Autodesk Inventor part; units mm, degrees
(part 4 of 4)
sketch "Sketch14" plane through (0, 0, 3) normal (0, 0, 1) x (1, 0, 0)
  line L0 (-25.3933, -129) -> (-25.3933, -146.5) projected
  line L1 (-25.3933, -146.5) -> (23.6067, -146.5) projected
  line L2 (23.6067, -146.5) -> (23.6067, -129) projected
  line L3 (23.6067, -129) -> (100.5, -129) projected
  line L4 (100.5, -129) -> (100.5, 184.5) projected
  line L5 (100.5, 184.5) -> (81, 184.5) projected
  line L6 (81, 184.5) -> (81, 215) projected
  line L7 (81, 215) -> (-78, 215) projected
  line L8 (-78, 215) -> (-78, 46.0635) projected
  line L9 (-78, 46.0635) -> (-75, 46.0635) projected
  line L10 (-75, 46.0635) -> (-75, 40.8932) projected
  line L11 (-75, 40.8932) -> (-78, 40.8932) projected
  line L12 (-78, 40.8932) -> (-78, 30.6062) projected
  line L13 (-78, 30.6062) -> (-75, 30.6062) projected
  line L14 (-75, 30.6062) -> (-75, 20.5478) projected
  line L15 (-75, 20.5478) -> (-78, 20.5478) projected
  line L16 (-78, 20.5478) -> (-78, 10.2608) projected
  line L17 (-78, 10.2608) -> (-75, 10.2608) projected
  line L18 (-75, 10.2608) -> (-75, -0.1068) projected
  line L19 (-75, -0.1068) -> (-78, -0.1068) projected
  line L20 (-78, -0.1068) -> (-78, -10.3938) projected
  line L21 (-78, -10.3938) -> (-75, -10.3938) projected
  line L22 (-75, -10.3938) -> (-75, -20.4522) projected
  line L23 (-75, -20.4522) -> (-78, -20.4522) projected
  line L24 (-78, -20.4522) -> (-78, -30.7392) projected
  line L25 (-78, -30.7392) -> (-75, -30.7392) projected
  line L26 (-75, -30.7392) -> (-75, -41.1068) projected
  line L27 (-75, -41.1068) -> (-78, -41.1068) projected
  line L28 (-78, -41.1068) -> (-78, -51.3938) projected
  line L29 (-78, -51.3938) -> (-75, -51.3938) projected
  line L30 (-75, -51.3938) -> (-75, -61.4522) projected
  line L31 (-75, -61.4522) -> (-78, -61.4522) projected
  line L32 (-78, -61.4522) -> (-78, -71.7392) projected
  line L33 (-78, -71.7392) -> (-75, -71.7392) projected
  line L34 (-75, -71.7392) -> (-75, -82.1068) projected
  line L35 (-75, -82.1068) -> (-78, -82.1068) projected
  line L36 (-78, -82.1068) -> (-78, -92.3938) projected
  line L37 (-78, -92.3938) -> (-75, -92.3938) projected
  line L38 (-75, -92.3938) -> (-75, -102.4522) projected
  line L39 (-75, -102.4522) -> (-78, -102.4522) projected
  line L40 (-78, -102.4522) -> (-78, -112.7392) projected
  line L41 (-78, -112.7392) -> (-75, -112.7392) projected
  line L42 (-75, -112.7392) -> (-75, -129) projected
  line L43 (-75, -129) -> (-25.3933, -129) projected
  arc A0 (46.9188, 54.6398) -> (53.7912, 60.27) centre (23.569, 90.1509) ccw projected
  arc A1 (35.9306, 51.3509) -> (46.9188, 54.6398) centre (35.9306, 71.3509) ccw projected
  line L44 (35.9306, 51.3509) -> (11.2074, 51.3509) projected
  arc A2 (0.2192, 54.6398) -> (11.2074, 51.3509) centre (11.2074, 71.3509) ccw projected
  arc A3 (-6.6532, 60.27) -> (0.2192, 54.6398) centre (23.569, 90.1509) ccw projected
  arc A4 (-12.431, 74.3316) -> (-6.6532, 60.27) centre (7.569, 74.3316) ccw projected
  line L45 (-12.431, 74.3316) -> (-12.431, 105.9702) projected
  arc A5 (-6.6532, 120.0317) -> (-12.431, 105.9702) centre (7.569, 105.9702) ccw projected
  arc A6 (0.2192, 125.662) -> (-6.6532, 120.0317) centre (23.569, 90.1509) ccw projected
  arc A7 (11.2074, 128.9509) -> (0.2192, 125.662) centre (11.2074, 108.9509) ccw projected
  line L46 (11.2074, 128.9509) -> (35.9306, 128.9509) projected
  arc A8 (46.9188, 125.662) -> (35.9306, 128.9509) centre (35.9306, 108.9509) ccw projected
  arc A9 (53.7912, 120.0317) -> (46.9188, 125.662) centre (23.569, 90.1509) ccw projected
  arc A10 (59.569, 105.9702) -> (53.7912, 120.0317) centre (39.569, 105.9702) ccw projected
  line L47 (59.569, 105.9702) -> (59.569, 74.3316) projected
  arc A11 (53.7912, 60.27) -> (59.569, 74.3316) centre (39.569, 74.3316) ccw projected
  circle A12 centre (-12.181, 208.9009) radius 1.2 projected
  circle A13 centre (59.319, 137.4009) radius 1.2 projected
  circle A14 centre (-12.181, 137.4009) radius 1.2 projected
  circle A15 centre (59.319, 54.4009) radius 1.2 projected
  circle A16 centre (-12.181, 125.9009) radius 1.2 projected
  circle A17 centre (59.319, 125.9009) radius 1.2 projected
  circle A18 centre (59.319, 208.9009) radius 1.2 projected
  circle A19 centre (-12.181, 54.4009) radius 1.2 projected
  arc A20 (46.9188, 137.6398) -> (53.7912, 143.27) centre (23.569, 173.1509) ccw projected
  arc A21 (35.9306, 134.3509) -> (46.9188, 137.6398) centre (35.9306, 154.3509) ccw projected
  line L48 (35.9306, 134.3509) -> (11.2074, 134.3509) projected
  arc A22 (0.2192, 137.6398) -> (11.2074, 134.3509) centre (11.2074, 154.3509) ccw projected
  arc A23 (-6.6532, 143.27) -> (0.2192, 137.6398) centre (23.569, 173.1509) ccw projected
  arc A24 (-12.431, 157.3316) -> (-6.6532, 143.27) centre (7.569, 157.3316) ccw projected
  line L49 (-12.431, 157.3316) -> (-12.431, 188.9702) projected
  arc A25 (-6.6532, 203.0317) -> (-12.431, 188.9702) centre (7.569, 188.9702) ccw projected
  arc A26 (0.2192, 208.662) -> (-6.6532, 203.0317) centre (23.569, 173.1509) ccw projected
  arc A27 (11.2074, 211.9509) -> (0.2192, 208.662) centre (11.2074, 191.9509) ccw projected
  line L50 (11.2074, 211.9509) -> (35.9306, 211.9509) projected
  arc A28 (46.9188, 208.662) -> (35.9306, 211.9509) centre (35.9306, 191.9509) ccw projected
  arc A29 (53.7912, 203.0317) -> (46.9188, 208.662) centre (23.569, 173.1509) ccw projected
  arc A30 (59.569, 188.9702) -> (53.7912, 203.0317) centre (39.569, 188.9702) ccw projected
  line L51 (59.569, 188.9702) -> (59.569, 157.3316) projected
  arc A31 (53.7912, 143.27) -> (59.569, 157.3316) centre (39.569, 157.3316) ccw projected
  circle A32 centre (90.5, 174.5) radius 2.25 projected
  circle A33 centre (90.5, 131.8987) radius 2.25 projected
  circle A34 centre (90.5, 58.3987) radius 2.25 projected
  circle A35 centre (90.5, -117.6237) radius 2.25 projected
  circle A36 centre (-17.8933, -140) radius 2.25 projected
  circle A37 centre (16.1067, -140) radius 2.25 projected
  line L52 (-58.9404, 10.4643) -> (-58.9404, 20.3443) projected
  arc A38 (-55.9404, 23.3443) -> (-58.9404, 20.3443) centre (-55.9404, 20.3443) ccw projected
  line L53 (-55.9404, 23.3443) -> (31.7396, 23.3443) projected
  arc A39 (34.7396, 20.3443) -> (31.7396, 23.3443) centre (31.7396, 20.3443) ccw projected
  line L54 (34.7396, 20.3443) -> (34.7396, 10.4643) projected
  arc A40 (31.7396, 7.4643) -> (34.7396, 10.4643) centre (31.7396, 10.4643) ccw projected
  line L55 (31.7396, 7.4643) -> (-55.9404, 7.4643) projected
  arc A41 (-58.9404, 10.4643) -> (-55.9404, 7.4643) centre (-55.9404, 10.4643) ccw projected
  line L56 (-58.9404, 30.8097) -> (-58.9404, 40.6897) projected
  arc A42 (-55.9404, 43.6897) -> (-58.9404, 40.6897) centre (-55.9404, 40.6897) ccw projected
  line L57 (-55.9404, 43.6897) -> (31.7396, 43.6897) projected
  arc A43 (34.7396, 40.6897) -> (31.7396, 43.6897) centre (31.7396, 40.6897) ccw projected
  line L58 (34.7396, 40.6897) -> (34.7396, 30.8097) projected
  arc A44 (31.7396, 27.8097) -> (34.7396, 30.8097) centre (31.7396, 30.8097) ccw projected
  line L59 (31.7396, 27.8097) -> (-55.9404, 27.8097) projected
  arc A45 (-58.9404, 30.8097) -> (-55.9404, 27.8097) centre (-55.9404, 30.8097) ccw projected
  arc A46 (-55.9404, 2.9989) -> (-58.9404, -0.0011) centre (-55.9404, -0.0011) ccw projected
  line L60 (-55.9404, 2.9989) -> (31.7396, 2.9989) projected
  arc A47 (34.7396, -0.0011) -> (31.7396, 2.9989) centre (31.7396, -0.0011) ccw projected
  line L61 (34.7396, -0.0011) -> (34.7396, -9.8811) projected
  arc A48 (31.7396, -12.8811) -> (34.7396, -9.8811) centre (31.7396, -9.8811) ccw projected
  line L62 (31.7396, -12.8811) -> (-55.9404, -12.8811) projected
  arc A49 (-58.9404, -9.8811) -> (-55.9404, -12.8811) centre (-55.9404, -9.8811) ccw projected
  line L63 (-58.9404, -9.8811) -> (-58.9404, -0.0011) projected
  arc A50 (-55.9404, -37.6919) -> (-58.9404, -40.6919) centre (-55.9404, -40.6919) ccw projected
  line L64 (-55.9404, -37.6919) -> (31.7396, -37.6919) projected
  arc A51 (34.7396, -40.6919) -> (31.7396, -37.6919) centre (31.7396, -40.6919) ccw projected
  line L65 (34.7396, -40.6919) -> (34.7396, -50.5719) projected
  arc A52 (31.7396, -53.5719) -> (34.7396, -50.5719) centre (31.7396, -50.5719) ccw projected
  line L66 (31.7396, -53.5719) -> (-55.9404, -53.5719) projected
  arc A53 (-58.9404, -50.5719) -> (-55.9404, -53.5719) centre (-55.9404, -50.5719) ccw projected
  line L67 (-58.9404, -50.5719) -> (-58.9404, -40.6919) projected
  line L68 (-55.9404, -58.0373) -> (31.7396, -58.0373) projected
  arc A54 (34.7396, -61.0373) -> (31.7396, -58.0373) centre (31.7396, -61.0373) ccw projected
  line L69 (34.7396, -61.0373) -> (34.7396, -70.9173) projected
  arc A55 (31.7396, -73.9173) -> (34.7396, -70.9173) centre (31.7396, -70.9173) ccw projected
  line L70 (31.7396, -73.9173) -> (-55.9404, -73.9173) projected
  arc A56 (-58.9404, -70.9173) -> (-55.9404, -73.9173) centre (-55.9404, -70.9173) ccw projected
  line L71 (-58.9404, -70.9173) -> (-58.9404, -61.0373) projected
  arc A57 (-55.9404, -58.0373) -> (-58.9404, -61.0373) centre (-55.9404, -61.0373) ccw projected
  line L72 (31.7396, -33.2265) -> (-55.9404, -33.2265) projected
  arc A58 (-58.9404, -30.2265) -> (-55.9404, -33.2265) centre (-55.9404, -30.2265) ccw projected
  line L73 (-58.9404, -30.2265) -> (-58.9404, -20.3465) projected
  arc A59 (-55.9404, -17.3465) -> (-58.9404, -20.3465) centre (-55.9404, -20.3465) ccw projected
  line L74 (-55.9404, -17.3465) -> (31.7396, -17.3465) projected
  arc A60 (34.7396, -20.3465) -> (31.7396, -17.3465) centre (31.7396, -20.3465) ccw projected
  line L75 (34.7396, -20.3465) -> (34.7396, -30.2265) projected
  arc A61 (31.7396, -33.2265) -> (34.7396, -30.2265) centre (31.7396, -30.2265) ccw projected
  arc A62 (34.7396, -81.3827) -> (31.7396, -78.3827) centre (31.7396, -81.3827) ccw projected
  line L76 (34.7396, -81.3827) -> (34.7396, -91.2627) projected
  arc A63 (31.7396, -94.2627) -> (34.7396, -91.2627) centre (31.7396, -91.2627) ccw projected
  line L77 (31.7396, -94.2627) -> (-55.9404, -94.2627) projected
  arc A64 (-58.9404, -91.2627) -> (-55.9404, -94.2627) centre (-55.9404, -91.2627) ccw projected
  line L78 (-58.9404, -91.2627) -> (-58.9404, -81.3827) projected
  arc A65 (-55.9404, -78.3827) -> (-58.9404, -81.3827) centre (-55.9404, -81.3827) ccw projected
  line L79 (-55.9404, -78.3827) -> (31.7396, -78.3827) projected
  arc A66 (31.7396, -114.6081) -> (34.7396, -111.6081) centre (31.7396, -111.6081) ccw projected
  line L80 (31.7396, -114.6081) -> (-55.9404, -114.6081) projected
  arc A67 (-58.9404, -111.6081) -> (-55.9404, -114.6081) centre (-55.9404, -111.6081) ccw projected
  line L81 (-58.9404, -111.6081) -> (-58.9404, -101.7281) projected
  arc A68 (-55.9404, -98.7281) -> (-58.9404, -101.7281) centre (-55.9404, -101.7281) ccw projected
  line L82 (-55.9404, -98.7281) -> (31.7396, -98.7281) projected
  arc A69 (34.7396, -101.7281) -> (31.7396, -98.7281) centre (31.7396, -101.7281) ccw projected
  line L83 (34.7396, -101.7281) -> (34.7396, -111.6081) projected
  line L84 (-69.3194, 50.0635) -> (-69.3194, 207.0635) projected
  arc A70 (-68.3194, 208.0635) -> (-69.3194, 207.0635) centre (-68.3194, 207.0635) ccw projected
  line L85 (-68.3194, 208.0635) -> (-25.6194, 208.0635) projected
  arc A71 (-24.6194, 207.0635) -> (-25.6194, 208.0635) centre (-25.6194, 207.0635) ccw projected
  line L86 (-24.6194, 207.0635) -> (-24.6194, 50.0635) projected
  arc A72 (-25.6194, 49.0635) -> (-24.6194, 50.0635) centre (-25.6194, 50.0635) ccw projected
  line L87 (-25.6194, 49.0635) -> (-68.3194, 49.0635) projected
  arc A73 (-69.3194, 50.0635) -> (-68.3194, 49.0635) centre (-68.3194, 50.0635) ccw projected
  line L88 (64, 48.3987) -> (64, -109.7094) projected
  arc A74 (63.7071, -110.4166) -> (64, -109.7094) centre (63, -109.7094) ccw projected
  line L89 (63.7071, -110.4166) -> (59.2929, -114.8308) projected
  arc A75 (58.5858, -115.1237) -> (59.2929, -114.8308) centre (58.5858, -114.1237) ccw projected
  line L90 (58.5858, -115.1237) -> (43.2196, -115.1237) projected
  arc A76 (42.2196, -114.1237) -> (43.2196, -115.1237) centre (43.2196, -114.1237) ccw projected
  line L91 (42.2196, -114.1237) -> (42.2196, -104.6674) projected
  arc A77 (42.2196, -104.6674) -> (40.773, -102.7455) centre (40.2196, -104.6674) ccw projected
  arc A78 (39.7673, -102.1811) -> (40.773, -102.7455) centre (41.4696, -100.3262) ccw projected
  arc A79 (39.1196, -100.7076) -> (39.7673, -102.1811) centre (41.1196, -100.7076) ccw projected
  line L92 (39.1196, -100.7076) -> (39.1196, -95.7515) projected
  arc A80 (39.7673, -94.2779) -> (39.1196, -95.7515) centre (41.1196, -95.7515) ccw projected
  arc A81 (39.937, -94.1354) -> (39.7673, -94.2779) centre (41.4696, -96.1328) ccw projected
  arc A82 (39.937, -94.1354) -> (40.7196, -92.5486) centre (38.7196, -92.5486) ccw projected
  line L93 (40.7196, -92.5486) -> (40.7196, -83.4104) projected
  arc A83 (40.7196, -83.4104) -> (39.937, -81.8236) centre (38.7196, -83.4104) ccw projected
  arc A84 (39.7673, -81.6811) -> (39.937, -81.8236) centre (41.4696, -79.8262) ccw projected
  arc A85 (39.1196, -80.2076) -> (39.7673, -81.6811) centre (41.1196, -80.2076) ccw projected
  line L94 (39.1196, -80.2076) -> (39.1196, -75.2515) projected
  arc A86 (39.7673, -73.7779) -> (39.1196, -75.2515) centre (41.1196, -75.2515) ccw projected
  arc A87 (39.937, -73.6354) -> (39.7673, -73.7779) centre (41.4696, -75.6328) ccw projected
  arc A88 (39.937, -73.6354) -> (40.7196, -72.0486) centre (38.7196, -72.0486) ccw projected
  line L95 (40.7196, -72.0486) -> (40.7196, -62.9104) projected
  arc A89 (40.7196, -62.9104) -> (39.937, -61.3236) centre (38.7196, -62.9104) ccw projected
  arc A90 (39.7673, -61.1811) -> (39.937, -61.3236) centre (41.4696, -59.3262) ccw projected
  arc A91 (39.1196, -59.7076) -> (39.7673, -61.1811) centre (41.1196, -59.7076) ccw projected
  line L96 (39.1196, -59.7076) -> (39.1196, -54.7515) projected
  arc A92 (39.7673, -53.2779) -> (39.1196, -54.7515) centre (41.1196, -54.7515) ccw projected
  arc A93 (39.937, -53.1354) -> (39.7673, -53.2779) centre (41.4696, -55.1328) ccw projected
  arc A94 (39.937, -53.1354) -> (40.7196, -51.5486) centre (38.7196, -51.5486) ccw projected
  line L97 (40.7196, -51.5486) -> (40.7196, -42.4104) projected
  arc A95 (40.7196, -42.4104) -> (39.937, -40.8236) centre (38.7196, -42.4104) ccw projected
  arc A96 (39.7673, -40.6811) -> (39.937, -40.8236) centre (41.4696, -38.8262) ccw projected
  arc A97 (39.1196, -39.2076) -> (39.7673, -40.6811) centre (41.1196, -39.2076) ccw projected
  line L98 (39.1196, -39.2076) -> (39.1196, -34.2515) projected
  arc A98 (39.7673, -32.7779) -> (39.1196, -34.2515) centre (41.1196, -34.2515) ccw projected
  arc A99 (39.937, -32.6354) -> (39.7673, -32.7779) centre (41.4696, -34.6328) ccw projected
  arc A100 (39.937, -32.6354) -> (40.7196, -31.0486) centre (38.7196, -31.0486) ccw projected
  line L99 (40.7196, -31.0486) -> (40.7196, -21.9104) projected
  arc A101 (40.7196, -21.9104) -> (39.937, -20.3236) centre (38.7196, -21.9104) ccw projected
  arc A102 (39.7673, -20.1811) -> (39.937, -20.3236) centre (41.4696, -18.3262) ccw projected
  arc A103 (39.1196, -18.7076) -> (39.7673, -20.1811) centre (41.1196, -18.7076) ccw projected
  line L100 (39.1196, -18.7076) -> (39.1196, -13.7515) projected
  arc A104 (39.7673, -12.2779) -> (39.1196, -13.7515) centre (41.1196, -13.7515) ccw projected
  arc A105 (39.937, -12.1354) -> (39.7673, -12.2779) centre (41.4696, -14.1328) ccw projected
  arc A106 (39.937, -12.1354) -> (40.7196, -10.5486) centre (38.7196, -10.5486) ccw projected
  line L101 (40.7196, -10.5486) -> (40.7196, -1.4104) projected
  arc A107 (40.7196, -1.4104) -> (39.937, 0.1764) centre (38.7196, -1.4104) ccw projected
  arc A108 (39.7673, 0.3189) -> (39.937, 0.1764) centre (41.4696, 2.1738) ccw projected
  arc A109 (39.1196, 1.7924) -> (39.7673, 0.3189) centre (41.1196, 1.7924) ccw projected
  line L102 (39.1196, 1.7924) -> (39.1196, 6.7485) projected
  arc A110 (39.7673, 8.2221) -> (39.1196, 6.7485) centre (41.1196, 6.7485) ccw projected
  arc A111 (39.937, 8.3646) -> (39.7673, 8.2221) centre (41.4696, 6.3672) ccw projected
  arc A112 (39.937, 8.3646) -> (40.7196, 9.9514) centre (38.7196, 9.9514) ccw projected
  line L103 (40.7196, 9.9514) -> (40.7196, 19.0896) projected
  arc A113 (40.7196, 19.0896) -> (39.937, 20.6764) centre (38.7196, 19.0896) ccw projected
  arc A114 (39.7673, 20.8189) -> (39.937, 20.6764) centre (41.4696, 22.6738) ccw projected
  arc A115 (39.1196, 22.2924) -> (39.7673, 20.8189) centre (41.1196, 22.2924) ccw projected
  line L104 (39.1196, 22.2924) -> (39.1196, 27.2485) projected
  arc A116 (39.7673, 28.7221) -> (39.1196, 27.2485) centre (41.1196, 27.2485) ccw projected
  arc A117 (39.937, 28.8646) -> (39.7673, 28.7221) centre (41.4696, 26.8672) ccw projected
  arc A118 (39.937, 28.8646) -> (40.7196, 30.4514) centre (38.7196, 30.4514) ccw projected
  line L105 (40.7196, 30.4514) -> (40.7196, 39.5896) projected
  arc A119 (40.7196, 39.5896) -> (39.937, 41.1764) centre (38.7196, 39.5896) ccw projected
  arc A120 (39.7673, 41.3189) -> (39.937, 41.1764) centre (41.4696, 43.1738) ccw projected
  arc A121 (39.1196, 42.7924) -> (39.7673, 41.3189) centre (41.1196, 42.7924) ccw projected
  line L106 (39.1196, 42.7924) -> (39.1196, 47.7485) projected
  arc A122 (39.7673, 49.2221) -> (39.1196, 47.7485) centre (41.1196, 47.7485) ccw projected
  arc A123 (43.3362, 49.0566) -> (39.7673, 49.2221) centre (41.4696, 47.3672) ccw projected
  arc A124 (43.3362, 49.0566) -> (44.819, 48.3987) centre (44.819, 50.3987) ccw projected
  line L107 (44.819, 48.3987) -> (64, 48.3987) projected
  point P0 (0, 0)
extrude "Extrusion14" add sketch "Sketch14" against normal up to surface (3 mm away) contours A1 L44 A2 A3 A4 L45 A5 A6 A7 L46 A8 A9 A10 L47 A11 A0 | A12 | A13 | A14 | A15 | A16 | A17 | A18 | A19 | A21 L48 A22 A23 A24 L49 A25 A26 A27 L50 A28 A29 A30 L51 A31 A20
sketch "Sketch15" plane through (0, 0, 3) normal (0, 0, 1) x (1, 0, 0)
  arc A0 (58.1623, 92.1588) -> (63.9401, 106.2204) centre (43.9401, 106.2204) ccw
  line L0 (40.3017, 83.2397) -> (15.5785, 83.2397)
  arc A1 (40.3017, 83.2397) -> (51.2899, 86.5286) centre (40.3017, 103.2397) ccw
  circle A2 centre (63.6901, 86.2897) radius 1.2
  line L1 (63.9401, 137.859) -> (63.9401, 106.2204)
  circle A3 centre (-7.8099, 157.7897) radius 1.2
  arc A4 (15.5785, 160.8397) -> (4.5903, 157.5508) centre (15.5785, 140.8397) ccw
  line L2 (15.5785, 160.8397) -> (40.3017, 160.8397)
  arc A5 (51.2899, 157.5508) -> (40.3017, 160.8397) centre (40.3017, 140.8397) ccw
  arc A6 (4.5903, 157.5508) -> (-2.2821, 151.9205) centre (27.9401, 122.0397) ccw
  circle A7 centre (63.6901, 157.7897) radius 1.2
  arc A8 (58.1623, 151.9205) -> (51.2899, 157.5508) centre (27.9401, 122.0397) ccw
  arc A9 (63.9401, 137.859) -> (58.1623, 151.9205) centre (43.9401, 137.859) ccw
  arc A10 (-2.2821, 151.9205) -> (-8.0599, 137.859) centre (11.9401, 137.859) ccw
  line L3 (-8.0599, 106.2204) -> (-8.0599, 137.859)
  arc A11 (-8.0599, 106.2204) -> (-2.2821, 92.1588) centre (11.9401, 106.2204) ccw
  arc A12 (4.5903, 86.5286) -> (15.5785, 83.2397) centre (15.5785, 103.2397) ccw
  arc A13 (-2.2821, 92.1588) -> (4.5903, 86.5286) centre (27.9401, 122.0397) ccw
  circle A14 centre (-7.8099, 86.2897) radius 1.2
  arc A15 (51.2899, 86.5286) -> (58.1623, 92.1588) centre (27.9401, 122.0397) ccw
  line L4 (17.3401, 185.8) -> (38.5401, 185.8)
  line L5 (41.5401, 188.8) -> (41.5401, 202)
  line L6 (38.5401, 205) -> (17.3401, 205)
  line L7 (14.3401, 202) -> (14.3401, 188.8)
  line L8 (14.3401, 185.8) -> (41.5401, 205) construction
  line L9 (41.5401, 185.8) -> (14.3401, 205) construction
  circle A16 centre (7.9401, 195.4) radius 3.615
  circle A17 centre (47.9401, 195.4) radius 3.615
  arc A18 (38.5401, 185.8) -> (41.5401, 188.8) centre (38.5401, 188.8) ccw
  arc A19 (14.3401, 188.8) -> (17.3401, 185.8) centre (17.3401, 188.8) ccw
  arc A20 (17.3401, 205) -> (14.3401, 202) centre (17.3401, 202) ccw
  arc A21 (41.5401, 202) -> (38.5401, 205) centre (38.5401, 202) ccw
  line L10 (81, 215) -> (-78, 215) projected
  line L11 (-24.6194, 207.0635) -> (-24.6194, 50.0635) projected
  point P0 (0, 0)
  point P1 (27.9401, 195.4)
  dimension "d120" = 2.4
  dimension "d121" = 20
  dimension "d122" = 42.5
  dimension "d123" = 42.5
  dimension "d124" = 42.5
  dimension "d125" = 42.5
  dimension "d126" = 72
  dimension "d127" = 77.6
  dimension "d130" = 22.9807
  dimension "d131" = 54.6193
  dimension "d132" = 0.25
  dimension "d133" = 3.05
  dimension "d134" = 0.25
  dimension "d135" = 74.55
  dimension "d136" = 5.7778
  dimension "d137" = 5.7778
  dimension "d138" = 12.6502
  dimension "d139" = 12.6502
  dimension "d140" = 36
  dimension "d141" = 38.8
  dimension "d142" = 71.75
  dimension "d143" = 3.05
  dimension "d144" = 71.75
  dimension "d145" = 74.55
  dimension "d146" = 27.2
  dimension "d147" = 19.2
  dimension "d148" = 9.6
  dimension "d149" = 20
  dimension "d152" = 40
  dimension "d157" = 3
  dimension "d158" = 10
  dimension "d174" = 52.5595
  dimension "d175" = 52.5595
  constraints: 32 point on circle, 24 tangent, 22 centre point, 20 end point, 13 equal radius, 8 point on line, 4 parallel, 3 horizontal, 2 midpoint, 1 perpendicular, 1 vertical, 2 other
  measures "d120" diameter of A7
  measures "d121" radius of A9
  measures "d122" radius of A15
  measures "d123" radius of A8
  measures "d124" radius of A13
  measures "d125" radius of A6
  measures "d126" distance between parallel lines of L1 L3
  measures "d127" distance between parallel lines of L2 L0
  measures "d130" distance from line of L1.start L2
  measures "d131" distance from line of L1.end L2
  measures "d132" distance from line of A7.centre L1
  measures "d133" distance from line of A7.centre L2
  measures "d134" distance from line of A2.centre L1
  measures "d135" distance from line of A2.centre L2
  measures "d136" distance from line of A9.end L1
  measures "d137" distance from line of A0.start L1
  measures "d138" distance from line of A8.end L1
  measures "d139" distance from line of A1.end L1
  measures "d140" distance from line of A13.centre L1
  measures "d141" distance from line of A13.centre L2
  measures "d142" distance from line of A3.centre L1
  measures "d143" distance from line of A3.centre L2
  measures "d144" distance from line of A14.centre L1
  measures "d145" distance from line of A14.centre L2
  measures "d146" distance between parallel lines of L5 L7
  measures "d147" distance between parallel lines of L6 L4
  measures "d148" distance from line of L6 A16.centre
  measures "d149" distance of point (27.94, 195.4) A16.centre
  measures "d152" distance of A16.centre A17.centre
  measures "d157" radius of A18
  measures "d158" distance between parallel lines of L10 L6
  measures "d174" distance from line of A15.centre L11
  measures "d175" distance from line of point (27.94, 195.4) L11
extrude "Extrusion15" cut sketch "Sketch15" against normal up to surface (3 mm away)
sketch "Sketch16" plane through (0, 0, 3) normal (0, 0, 1) x (1, 0, 0)
  line L0 (23.6067, -129) -> (100.5, -129) projected
  line L1 (100.5, -129) -> (100.5, 184.5) projected
  line L2 (100.5, 184.5) -> (81, 184.5) projected
  line L3 (81, 184.5) -> (81, 215) projected
  line L4 (81, -129) -> (81, -98.5)
  line L5 (81, -98.5) -> (100.5, -98.5)
  circle A0 centre (90.5, -117.6237) radius 2.25 projected
  circle A1 centre (90.5, 174.5) radius 2.25 projected
  circle A2 centre (90.5, -88.5) radius 2.25
  point P0 (0, 0)
  dimension "d161" = 30.5
  dimension "d162" = 10
  dimension "d163" = 4.5
  dimension "d164" = 10
  dimension "d165" = 4.5
  dimension "d166" = 10
  dimension "d167" = 10
  dimension "d172" = 19.5
  dimension "d173" = 19.5
  constraints: 4 end point, 2 point on line, 1 centre point, 1 perpendicular, 1 vertical
  measures "d161" distance of L4.start L4.end
  measures "d162" distance from line of L2 A1.centre
  measures "d163" diameter of A1
  measures "d164" distance from line of L1 A1.centre
  measures "d165" diameter of A2
  measures "d166" distance from line of L5 A2.centre
  measures "d167" distance from line of L1 A2.centre
  measures "d172" distance of L1.end L2.end
  measures "d173" distance of L4.end L5.end
extrude "Extrusion17" cut sketch "Sketch16" against normal up to surface (3 mm away) contours L4 L5 L1 L0 | A2
sketch "Sketch17" plane through (0, 0, 3) normal (0, 0, 1) x (1, 0, 0)
  line L0 (23.6067, -129) -> (23.6067, -146.5) projected
  line L1 (23.6067, -146.5) -> (48.9997, -146.5)
  line L2 (48.9997, -146.5) -> (48.9997, -129)
  line L3 (48.9997, -129) -> (23.6067, -129)
  line L4 (23.6067, -129) -> (23.6067, -146.5)
  line L5 (81, -129) -> (81, -98.5) projected
  line L6 (-25.3933, -129) -> (-25.3933, -146.5) projected
  line L7 (-25.3933, -129) -> (-75, -129) projected
  line L8 (-25.3933, -146.5) -> (-44.0003, -146.5)
  line L9 (-44.0003, -146.5) -> (-44.0003, -129)
  line L10 (-44.0003, -129) -> (-25.3933, -129)
  line L11 (-25.3933, -129) -> (-25.3933, -146.5)
  line L12 (-44.0003, 215) -> (48.9997, 215)
  line L13 (48.9997, 215) -> (48.9997, 232.5)
  line L14 (48.9997, 232.5) -> (-44.0003, 232.5)
  line L15 (-44.0003, 232.5) -> (-44.0003, 215)
  line L16 (81, 215) -> (81, 184.5) projected
  line L17 (-78, 215) -> (81, 215) projected
  point P0 (0, 0)
  dimension "d177" = 25.393
  dimension "d179" = 18.607
  dimension "d182" = 93
  dimension "d183" = 17.5
  dimension "d184" = 32.0003
  dimension "d185" = 93
  dimension "d186" = 17.5
  dimension "d187" = 32.0003
  constraints: 24 end point, 6 parallel, 3 horizontal, 3 perpendicular, 1 collinear, 1 point on line
  measures "d177" distance between parallel lines of L2 L4
  measures "d179" distance between parallel lines of L6 L9
  measures "d182" distance between parallel lines of L2 L9
  measures "d183" distance of L1.end L2.end
  measures "d184" distance between parallel lines of L5 L2
  measures "d185" distance of L13.end L14.end
  measures "d186" distance of L12.end L13.end
  measures "d187" distance between parallel lines of L16 L13
extrude "Extrusion19" add sketch "Sketch17" against normal up to surface (3 mm away)
sketch "Sketch18" plane through (0, 0, 0) normal (0, 0, -1) x (-1, 0, 0)
  circle A0 centre (17.8933, -140) radius 2.25 projected
  line L0 (-48.9997, -146.5) -> (44.0003, -146.5) projected
  line L1 (-48.9997, -129) -> (-48.9997, -146.5) projected
  circle A1 centre (-16.1067, -140) radius 2.25 projected
  circle A2 centre (17.8933, 226) radius 2.25
  circle A3 centre (-16.1067, 226) radius 2.25
  line L2 (-48.9997, 232.5) -> (-48.9997, 215) projected
  line L3 (44.0003, 232.5) -> (-48.9997, 232.5) projected
  point P0 (0, 0)
  dimension "d190" = 4.5
  dimension "d191" = 6.5
  dimension "d192" = 32.893
  dimension "d193" = 34
  dimension "d194" = 4.5
  dimension "d195" = 4.5
  dimension "d196" = 34
  dimension "d197" = 32.893
  dimension "d198" = 6.5
  dimension "d199" = 6.5
  constraints: 2 centre point
  measures "d190" diameter of A0
  measures "d191" distance from line of L0 A0.centre
  measures "d192" distance from line of L1 A1.centre
  measures "d193" distance of A0.centre A1.centre
  measures "d194" diameter of A3
  measures "d195" diameter of A2
  measures "d196" distance of A3.centre A2.centre
  measures "d197" distance from line of L2 A3.centre
  measures "d198" distance from line of L3 A3.centre
  measures "d199" distance from line of L3 A2.centre
extrude "Extrusion20" cut sketch "Sketch18" against normal up to surface (3 mm away) contours A2 | A3
sketch "Sketch19" plane through (0, 0, 0) normal (0, 0, -1) x (-1, 0, 0)
  line L0 (78, 46.0635) -> (78, 215) projected
  line L1 (78, 215) -> (95.5, 215)
  line L2 (95.5, 215) -> (95.5, 46.0635)
  line L3 (95.5, 46.0635) -> (78, 46.0635)
  line L4 (78, 46.0635) -> (78, 215)
  circle A0 centre (-90.5, 58.3987) radius 2.25 projected
  line L5 (-100.5, 184.5) -> (-100.5, -98.5) projected
  circle A1 centre (85.5, 66.0635) radius 2.25
  line L6 (78, 215) -> (78, 46.0635) projected
  line L7 (78, 184.5) -> (95.5, 184.5)
  line L8 (-81, 184.5) -> (-100.5, 184.5) projected
  line L9 (-48.9997, 215) -> (-81, 215) projected
  circle A2 centre (85.5, 174.5) radius 2.25
  circle A3 centre (-90.5, 174.5) radius 2.25 projected
  circle A4 centre (85.5, 120.2818) radius 2.25
  point P0 (0, 0)
  dimension "d202" = 17.5
  dimension "d203" = 4.5
  dimension "d204" = 10
  dimension "d205" = 4.5
  dimension "d206" = 10
  dimension "d207" = 30.5
  dimension "d208" = 30.5
  dimension "d209" = 4.5
  dimension "d210" = 10
  dimension "d211" = 10
  dimension "d212" = 10
  dimension "d213" = 4.5
  dimension "d214" = 10
  dimension "d215" = 20
  dimension "d216" = 108.4365
  dimension "d217" = 54.2182
  constraints: 10 end point, 3 centre point, 2 parallel, 2 perpendicular, 2 point on line, 1 horizontal
  measures "d202" distance between parallel lines of L0 L2
  measures "d203" diameter of A0
  measures "d204" distance from line of L5 A0.centre
  measures "d205" diameter of A1
  measures "d206" distance from line of L2 A1.centre
  measures "d207" distance between parallel lines of L8 L9
  measures "d208" distance between parallel lines of L1 L7
  measures "d209" diameter of A2
  measures "d210" distance from line of A2.centre L2
  measures "d211" distance from line of L8 A3.centre
  measures "d212" distance from line of L7 A2.centre
  measures "d213" diameter of A4
  measures "d214" distance from line of L2 A4.centre
  measures "d215" distance from line of L3 A1.centre
  measures "d216" distance of A2.centre A1.centre
  measures "d217" distance of A4.centre A1.centre
extrude "Extrusion21" add sketch "Sketch19" against normal up to surface (3 mm away) contours L0 L7 L2 L3
sketch "Sketch20" plane through (0, 0, 0) normal (0, 0, -1) x (-1, 0, 0)
  line L0 (-48.9997, -146.5) -> (44.0003, -146.5) projected
  circle A0 centre (17.8933, -140) radius 2.25 projected
  line L1 (-100.5, 184.5) -> (-100.5, -98.5) projected
  circle A1 centre (-90.5, -88.5) radius 2.25 projected
  line L2 (-100.5, -98.5) -> (-81, -98.5) projected
  line L3 (-81, 184.5) -> (-100.5, 184.5) projected
  line L4 (95.5, 46.0635) -> (95.5, 184.5) projected
  line L5 (75, 46.0635) -> (95.5, 46.0635) projected
  line L6 (95.5, 184.5) -> (78, 184.5) projected
  line L7 (-97, -98.5) -> (-97, 184.5)
  line L8 (92, 46.0635) -> (92, 184.5)
  point P0 (0, 0)
  point P1 (78, 40.8932)
  dimension "d220" = 6.5
  dimension "d221" = 10
  dimension "d222" = 3.5
  dimension "d223" = 3.5
  constraints: 4 end point, 4 point on line, 2 perpendicular
  measures "d220" distance from line of A0.centre L0
  measures "d221" distance from line of L1 A1.centre
  measures "d222" distance between parallel lines of L1 L7
  measures "d223" distance between parallel lines of L8 L4
extrude "Extrusion22" cut sketch "Sketch20" against normal up to surface (3 mm away) contours L3 L7 L2 L1 | L5 L8 L6 L4
equation "\"d20\" = d19"
equation "\"d27\" = d26"
equation "\"d28\" = d23"
equation "\"d29\" = d24"
equation "\"d42\" = d41"
equation "\"d43\" = d40"
equation "\"d50\" = d48"
equation "\"d51\" = d49"
equation "\"d52\" = d50"
equation "\"d54\" = d52"
body "Solid2"
